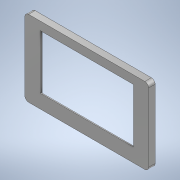
# Autodesk Inventor part: DisplayCover
Saved by Autodesk Inventor 2020 (Build 240168000, 168)
## iProperties
Created: 2021-05-02
Part Number: DisplayCover
Material: ABS Plastic
Document SubType Name: Modeling
Designer: 10300812
Density: 1.06 g/cm^3
Appearance: Anodized - Light Gray
Author: 10300812
Autodesk Inventor part; units mm, degrees
ref_plane "YZ Plane" through (0, 0, 0) normal (1, 0, 0) x (0, 1, 0)
ref_plane "XZ Plane" through (0, 0, 0) normal (0, 1, 0) x (-1, 0, 0)
ref_plane "XY Plane" through (0, 0, 0) normal (0, 0, 1) x (1, 0, 0)
sketch "Sketch1" plane through (0, 0, 0) normal (0, 0, 1) x (1, 0, 0)
  line L0 (-61, 40) -> (61, 40)
  line L1 (65, 36) -> (65, -36)
  line L2 (61, -40) -> (-61, -40)
  line L3 (-65, -36) -> (-65, 36)
  line L4 (-65, 40) -> (65, -40) construction
  line L5 (65, 40) -> (-65, -40) construction
  arc A0 (-61, 40) -> (-65, 36) centre (-61, 36) ccw
  arc A1 (-65, -36) -> (-61, -40) centre (-61, -36) ccw
  arc A2 (61, -40) -> (65, -36) centre (61, -36) ccw
  arc A3 (65, 36) -> (61, 40) centre (61, 36) ccw
  point P0 (0, 0)
  dimension "d0" = 130
  dimension "d1" = 80
  dimension "d2" = 4
  constraints: 12 end point, 8 point on circle, 8 point on line, 8 tangent, 4 centre point, 3 equal radius, 2 midpoint, 2 parallel, 1 horizontal, 1 perpendicular
  measures "d0" distance of L4.end L5.end
  measures "d1" distance of L5.start L4.end
  measures "d2" radius of A0
extrude "Extrusion1" add sketch "Sketch1" along normal blind 6.855
sketch "Sketch2" plane through (0, 0, 6.855) normal (0, 0, 1) x (1, 0, 0)
  line L0 (49.225, 31.315) -> (-48.825, 31.315) projected
  line L1 (-48.825, 31.315) -> (-48.825, -25.535) projected
  line L2 (-48.825, -25.535) -> (49.225, -25.535) projected
  line L3 (49.225, -25.535) -> (49.225, 31.315) projected
  point P0 (0, 0)
extrude "Extrusion2" cut sketch "Sketch2" against normal through all
sketch "Sketch3" plane through (0, 0, 0) normal (0, 0, -1) x (-1, 0, 0)
  line L0 (-52.95, -31.635) -> (-52.95, 31.69) projected
  line L1 (-51.025, 33.615) -> (50.55, 33.615) projected
  line L2 (50.55, 33.615) -> (50.747, 33.615) projected
  line L3 (50.747, 33.615) -> (51.1334, 33.5382) projected
  line L4 (51.1334, 33.5382) -> (51.4974, 33.3874) projected
  line L5 (51.4974, 33.3874) -> (51.8249, 33.1685) projected
  line L6 (51.8249, 33.1685) -> (52.1035, 32.8899) projected
  line L7 (52.1035, 32.8899) -> (52.3224, 32.5624) projected
  line L8 (52.3224, 32.5624) -> (52.4731, 32.1984) projected
  line L9 (52.4731, 32.1984) -> (52.55, 31.812) projected
  line L10 (52.55, 31.812) -> (52.55, 31.615) projected
  line L11 (52.55, 31.615) -> (52.55, -31.635) projected
  line L12 (52.55, -31.635) -> (52.55, -31.827) projected
  line L13 (52.55, -31.827) -> (52.4751, -32.2038) projected
  line L14 (52.4751, -32.2038) -> (52.3281, -32.5587) projected
  line L15 (52.3281, -32.5587) -> (52.1147, -32.878) projected
  line L16 (52.1147, -32.878) -> (51.843, -33.1497) projected
  line L17 (51.843, -33.1497) -> (51.5237, -33.3631) projected
  line L18 (51.5237, -33.3631) -> (51.1688, -33.5101) projected
  line L19 (51.1688, -33.5101) -> (50.7921, -33.585) projected
  line L20 (50.7921, -33.585) -> (50.6, -33.585) projected
  line L21 (50.6, -33.585) -> (-51, -33.585) projected
  line L22 (-52.95, -31.827) -> (-52.95, -31.635) projected
  line L23 (-52.8751, -32.2038) -> (-52.95, -31.827) projected
  line L24 (-52.7281, -32.5587) -> (-52.8751, -32.2038) projected
  line L25 (-52.5147, -32.878) -> (-52.7281, -32.5587) projected
  line L26 (-52.2431, -33.1497) -> (-52.5147, -32.878) projected
  line L27 (-51.9237, -33.3631) -> (-52.2431, -33.1497) projected
  line L28 (-51.5688, -33.5101) -> (-51.9237, -33.3631) projected
  line L29 (-51.1921, -33.585) -> (-51.5688, -33.5101) projected
  line L30 (-51, -33.585) -> (-51.1921, -33.585) projected
  line L31 (-51.2146, 33.615) -> (-51.025, 33.615) projected
  line L32 (-51.5865, 33.541) -> (-51.2146, 33.615) projected
  line L33 (-51.9368, 33.3959) -> (-51.5865, 33.541) projected
  line L34 (-52.2521, 33.1853) -> (-51.9368, 33.3959) projected
  line L35 (-52.5203, 32.9171) -> (-52.2521, 33.1853) projected
  line L36 (-52.7309, 32.6018) -> (-52.5203, 32.9171) projected
  line L37 (-52.876, 32.2515) -> (-52.7309, 32.6018) projected
  line L38 (-52.95, 31.8796) -> (-52.876, 32.2515) projected
  line L39 (-52.95, 31.69) -> (-52.95, 31.8796) projected
  line L40 (50.55, 34.615) -> (-51.025, 34.615)
  line L41 (-51.025, 34.615) -> (-51.3131, 34.615)
  line L42 (-51.3131, 34.615) -> (-51.8782, 34.5026)
  line L43 (-51.8782, 34.5026) -> (-52.4105, 34.2821)
  line L44 (-52.4105, 34.2821) -> (-52.8896, 33.962)
  line L45 (-52.8896, 33.962) -> (-53.297, 33.5546)
  line L46 (-53.297, 33.5546) -> (-53.6171, 33.0755)
  line L47 (-53.6171, 33.0755) -> (-53.8376, 32.5432)
  line L48 (-53.8376, 32.5432) -> (-53.95, 31.9781)
  line L49 (-53.95, 31.9781) -> (-53.95, 31.69)
  line L50 (-53.95, 31.69) -> (-53.95, -31.635)
  line L51 (-53.95, -31.635) -> (-53.95, -31.9255)
  line L52 (-53.95, -31.9255) -> (-53.8366, -32.4955)
  line L53 (-53.8366, -32.4955) -> (-53.6143, -33.0323)
  line L54 (-53.6143, -33.0323) -> (-53.2914, -33.5155)
  line L55 (-53.2914, -33.5155) -> (-52.8805, -33.9264)
  line L56 (-52.8805, -33.9264) -> (-52.3974, -34.2492)
  line L57 (-52.3974, -34.2492) -> (-51.8605, -34.4716)
  line L58 (-51.8605, -34.4716) -> (-51.2906, -34.585)
  line L59 (-51.2906, -34.585) -> (-51, -34.585)
  line L60 (-51, -34.585) -> (50.6, -34.585)
  line L61 (50.6, -34.585) -> (50.8905, -34.585)
  line L62 (50.8905, -34.585) -> (51.4605, -34.4716)
  line L63 (51.4605, -34.4716) -> (51.9973, -34.2492)
  line L64 (51.9973, -34.2492) -> (52.4805, -33.9264)
  line L65 (52.4805, -33.9264) -> (52.8914, -33.5155)
  line L66 (52.8914, -33.5155) -> (53.2143, -33.0323)
  line L67 (53.2143, -33.0323) -> (53.4366, -32.4955)
  line L68 (53.4366, -32.4955) -> (53.55, -31.9255)
  line L69 (53.55, -31.9255) -> (53.55, -31.635)
  line L70 (53.55, -31.635) -> (53.55, 31.615)
  line L71 (53.55, 31.615) -> (53.55, 31.9105)
  line L72 (53.55, 31.9105) -> (53.4347, 32.4901)
  line L73 (53.4347, 32.4901) -> (53.2086, 33.036)
  line L74 (53.2086, 33.036) -> (52.8803, 33.5274)
  line L75 (52.8803, 33.5274) -> (52.4624, 33.9453)
  line L76 (52.4624, 33.9453) -> (51.971, 34.2736)
  line L77 (51.971, 34.2736) -> (51.4251, 34.4997)
  line L78 (51.4251, 34.4997) -> (50.8455, 34.615)
  line L79 (50.8455, 34.615) -> (50.55, 34.615)
  point P0 (0, 0)
  dimension "d7" = 1
  constraints: 80 end point, 39 other
  measures "d7" distance between parallel lines of L1 L40
extrude "Extrusion3" cut sketch "Sketch3" against normal blind 5.855 contours L0 L39 L38 L37 L36 L35 L34 L33 L32 L31 L1 L2 L3 L4 L5 L6 L7 L8 L9 L10 L11 L12 L13 L14 L15 L16 L17 L18 L19 L20 L21 L30 L29 L28 L27 L26 L25 L24 L23 L22 | L79 L78 L77 L76 L75 L74 L73 L72 L71 L70 L69 L68 L67 L66 L65 L64 L63 L62 L61 L60 L59 L58 L57 L56 L55 L54 L53 L52 L51 L50 L49 L48 L47 L46 L45 L44 L43 L42 L41 L40
sketch "Sketch4" plane through (0, 0, 0) normal (0, 0, -1) x (-1, 0, 0)
  line L0 (-58.1378, 13.8535) -> (-62.7167, 13.8535)
  line L1 (-62.7167, 13.8535) -> (-62.7167, 7.4621)
  line L2 (-62.7167, 7.4621) -> (-58.1378, 7.4621)
  line L3 (-58.1378, 7.4621) -> (-58.1378, 13.8535)
  line L4 (-58.1378, 13.8535) -> (-62.7167, 7.4621) construction
  line L5 (-62.7167, 13.8535) -> (-58.1378, 7.4621) construction
  line L6 (-57.8993, -7.1808) -> (-62.9552, -7.1808)
  line L7 (-62.9552, -7.1808) -> (-62.9552, -13.763)
  line L8 (-62.9552, -13.763) -> (-57.8993, -13.763)
  line L9 (-57.8993, -13.763) -> (-57.8993, -7.1808)
  line L10 (-57.8993, -7.1808) -> (-62.9552, -13.763) construction
  line L11 (-62.9552, -7.1808) -> (-57.8993, -13.763) construction
  point P0 (0, 0)
  point P1 (-60.4272, 10.6578)
  point P2 (-60.4272, -10.4719)
  constraints: 24 end point, 4 midpoint, 4 parallel, 2 horizontal, 2 perpendicular
extrude "Extrusion4" cut sketch "Sketch4" against normal blind 3
sketch "Sketch5" plane through (0, 0, 0) normal (0, 0, -1) x (-1, 0, 0)
  circle A0 centre (61, 36) radius 1.625 projected
  circle A1 centre (61, -36) radius 1.625 projected
  circle A2 centre (-61, -36) radius 1.625 projected
  circle A3 centre (-61, 36) radius 1.625 projected
  point P0 (0, 0)
  constraints: 4 coincident
hole "Hole1" at (61, 36, 0) at (61, -36, 0) at (-61, 36, 0) at (-61, -36, 0) direction (0, 0, 1) diameter 2.459 depth 5.5 thread size "M3x0.5" class "6H" standard "ANSI Metric M Profile"
sketch "Sketch6" plane through (0, 0, 0) normal (0, 0, -1) x (-1, 0, 0)
  line L0 (50.8905, -34.585) -> (-51.2906, -34.585) projected
  line L1 (-51.2906, -34.585) -> (-0.2, -34.585)
  line L2 (-0.2, -34.585) -> (-0.2, -36.585)
  line L3 (-0.2, -36.585) -> (-51.2906, -36.585)
  line L4 (-51.2906, -36.585) -> (-51.2906, -34.585)
  point P0 (0, 0)
  dimension "d19" = 2
  constraints: 8 end point, 2 parallel, 1 horizontal, 1 perpendicular
  measures "d19" distance of L3.end L0.end
extrude "Extrusion5" cut sketch "Sketch6" against normal up to surface (5.855 mm away)
fillet "Fillet1" radius 2 2 edges at (0.2, -34.585, 2.9275) (51.2906, -34.585, 2.9275)
body "Solid1"
